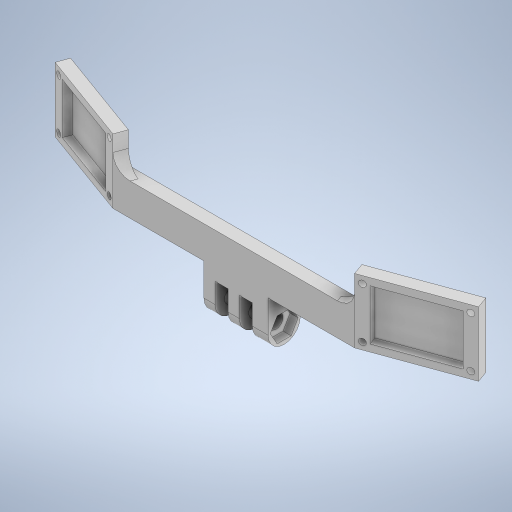
# Autodesk Inventor part: Camera dual mount
Saved by Autodesk Inventor 2024 (Build 280153000, 153)
## iProperties
Created: 2023-07-02
Part Number: Camera dual mount
Material: Generic
Document SubType Name: Modeling
Designer: TEST BENCH
Density: 1 g/cm^3
Appearance: Default
Author: TEST BENCH
Autodesk Inventor part; units mm, degrees
note: some values were not read from the file. Chosen so that the rebuilt part matches the saved one: edges of "Chamfer1".
ref_plane "YZ Plane" through (0, 0, 0) normal (1, 0, 0) x (0, 1, 0)
ref_plane "XZ Plane" through (0, 0, 0) normal (0, 1, 0) x (-1, 0, 0)
ref_plane "XY Plane" through (0, 0, 0) normal (0, 0, 1) x (1, 0, 0)
sketch "Sketch1" plane through (0, 0, 0) normal (0, 0, 1) x (1, 0, 0)
  line L0 (-32.5, 24) -> (32.5, 24)
  line L1 (32.5, 24) -> (32.5, 0)
  line L2 (32.5, 0) -> (-32.5, 0)
  line L3 (-32.5, 0) -> (-32.5, 24)
  point P0 (0, 0)
  dimension "d0" = 0
  dimension "d2" = 65
  dimension "d3" = 32.5
  dimension "d4" = 24
  constraints: 8 end point, 2 parallel, 1 horizontal, 1 perpendicular
  measures "d0" distance from line of L2 point (0, 0)
  measures "d2" distance between parallel lines of L1 L3
  measures "d3" distance from line of point (0, 0) L3
  measures "d4" distance between parallel lines of L2 L0
sketch "Sketch2" plane through (0, 0, 0) normal (0, 1, 0) x (-1, 0, 0)
  line L0 (28.9739, 0) -> (-28.9739, 0) construction
  line L1 (28.9739, 0) -> (51.5266, -8.2085)
  line L2 (51.5266, -8.2085) -> (52.5526, -5.3894)
  line L3 (52.5526, -5.3894) -> (30, 2.8191)
  line L4 (30, 2.8191) -> (28.9739, 0)
  line L5 (-28.9739, 0) -> (-51.5266, -8.2085)
  line L6 (-51.5266, -8.2085) -> (-52.5526, -5.3894)
  line L7 (-52.5526, -5.3894) -> (-30, 2.8191)
  line L8 (-30, 2.8191) -> (-28.9739, 0)
  line L9 (30, 2.8191) -> (-30, 2.8191)
  line L10 (-30, 2.8191) -> (-30, -0.3735)
  line L11 (-30, -0.3735) -> (30, -0.3735)
  line L12 (30, -0.3735) -> (30, 2.8191)
  point P0 (0, 0)
  point P1 (0, 0)
  point P2 (40.2503, -4.1042)
  point P3 (-30, -0.3735)
  dimension "d11" = 160
  dimension "d12" = 160
  dimension "d13" = 0
  dimension "d14" = 0
  dimension "d15" = 3
  dimension "d16" = 24
  dimension "d17" = 24
  dimension "d18" = 3
  dimension "d19" = 0
  dimension "d20" = 60
  constraints: 26 end point, 6 parallel, 3 perpendicular, 2 midpoint, 1 horizontal
  measures "d11" angle of L0 L1
  measures "d12" angle of L5 L0
  measures "d13" distance of point (0, 0) point (0, 0)
  measures "d14" distance of point (0, 0) point (0, 0)
  measures "d15" distance from line of point (40.25, -4.104) L3
  measures "d16" distance of L2.end L3.end
  measures "d17" distance of L6.end L7.end
  measures "d18" distance of L7.end L0.end
  measures "d19" distance from line of L1 L11.end
  measures "d20" distance of L3.end L7.end
extrude "Extrusion1" add sketch "Sketch2" along normal blind 16 contours L4 L12 L1 | L12 L3 L2 L1 | L10 L8 L5 | L5 L6 L7 L10
extrude "Extrusion2" add sketch "Sketch2" along normal blind 8 contours L1 L11 L5 L8 L9 L4
fillet "Fillet1" radius 4 2 edges at (-29.487, 8, 1.4095) (29.487, 8, 1.4095)
sketch "Sketch3" plane through (0, 0, 0) normal (0, -1, 0) x (1, 0, 0)
  line L0 (-25.7433, 2.8191) -> (25.7433, 2.8191) projected
  line L1 (-1.5, 2.8191) -> (1.5, 2.8191)
  line L2 (1.5, 2.8191) -> (1.5, -5.1809)
  line L3 (1.5, -5.1809) -> (-1.5, -5.1809)
  line L4 (-1.5, -5.1809) -> (-1.5, 2.8191)
  line L5 (-4.5, 2.8191) -> (-7.5, 2.8191)
  line L6 (-7.5, 2.8191) -> (-7.5, -5.1809)
  line L7 (-7.5, -5.1809) -> (-4.5, -5.1809)
  line L8 (-4.5, -5.1809) -> (-4.5, 2.8191)
  line L9 (4.5, 2.8191) -> (8.5, 2.8191)
  line L10 (8.5, 2.8191) -> (8.5, -5.1809)
  line L11 (8.5, -5.1809) -> (4.5, -5.1809)
  line L12 (4.5, -5.1809) -> (4.5, 2.8191)
  line L13 (8.5, -5.1809) -> (-7.5, -5.1809)
  line L14 (-7.5, -5.1809) -> (-7.5, 2.8191)
  line L15 (-7.5, 2.8191) -> (8.5, 2.8191)
  line L16 (8.5, 2.8191) -> (8.5, -5.1809)
  line L17 (-1.4, 2.8191) -> (1.4, 2.8191)
  line L18 (1.4, 2.8191) -> (1.4, -5.1809)
  line L19 (1.4, -5.1809) -> (-1.4, -5.1809)
  line L20 (-1.4, -5.1809) -> (-1.4, 2.8191)
  line L21 (-7.4, 2.8191) -> (-4.6, 2.8191)
  line L22 (-4.6, 2.8191) -> (-4.6, -5.1809)
  line L23 (-4.6, -5.1809) -> (-7.4, -5.1809)
  line L24 (-7.4, -5.1809) -> (-7.4, 2.8191)
  line L25 (4.6, 2.8191) -> (8.5, 2.8191)
  line L26 (8.5, 2.8191) -> (8.5, -5.1809)
  line L27 (8.5, -5.1809) -> (4.6, -5.1809)
  line L28 (4.6, -5.1809) -> (4.6, 2.8191)
  line L29 (-7.4, 2.8191) -> (-7.5, 2.8191)
  line L30 (-7.5, 2.8191) -> (-7.5, -5.1809)
  line L31 (-7.5, -5.1809) -> (-7.4, -5.1809)
  line L32 (-7.4, -5.1809) -> (-7.4, 2.8191)
  line L33 (-4.6, 2.8191) -> (-4.5, 2.8191)
  line L34 (-4.5, 2.8191) -> (-4.5, -5.1809)
  line L35 (-4.5, -5.1809) -> (-4.6, -5.1809)
  line L36 (-4.6, -5.1809) -> (-4.6, 2.8191)
  point P0 (0, 0)
  point P1 (0, -5.1809)
  point P2 (0, 2.8191)
  point P3 (-1.5, -1.1809)
  point P4 (4.5, -1.1809)
  point P5 (1.5, 2.8191)
  point P6 (8.5, 2.8191)
  dimension "d26" = 8
  dimension "d27" = 3
  dimension "d28" = 3
  dimension "d29" = 3
  dimension "d30" = 3
  dimension "d31" = 1.5
  dimension "d32" = 4
  dimension "d68" = 2.8
  dimension "d69" = 2.8
  dimension "d70" = 0.1
  dimension "d71" = 0.1
  dimension "d72" = 0.1
  constraints: 72 end point, 18 parallel, 9 horizontal, 9 perpendicular, 9 point on line, 4 midpoint, 1 collinear
  measures "d26" distance of point (0, -5.181) point (0, 2.819)
  measures "d27" distance from line of point (-1.5, -1.181) L2
  measures "d28" distance between parallel lines of L8 L6
  measures "d29" distance between parallel lines of L4 L8
  measures "d30" distance between parallel lines of L12 L2
  measures "d31" distance from line of point (0, 0) L4
  measures "d32" distance from line of point (4.5, -1.181) L10
  measures "d68" distance between parallel lines of L22 L24
  measures "d69" distance between parallel lines of L18 L20
  measures "d70" distance between parallel lines of L14 L24
  measures "d71" distance between parallel lines of L4 L20
  measures "d72" distance between parallel lines of L12 L28
extrude "Extrusion3" add sketch "Sketch3" along normal blind 3 contours L0 L22 L7 L24 | L0 L8 L7 L22 | L0 L4 L13 L8 | L0 L20 L3 L4 | L0 L18 L3 L20 | L0 L2 L3 L18 | L0 L12 L13 L2 | L0 L28 L11 L12 | L0 L10 L11 L28
extrude "Extrusion4" add sketch "Sketch3" along normal blind 12 contours L0 L22 L7 L24 | L0 L18 L3 L20 | L0 L10 L11 L28
fillet "Fillet2" radius 4 6 edges at (6.55, -12, 2.8191) (0, -12, 2.8191) (-6, -12, 2.8191) (-6, -12, -5.1809) (0, -12, -5.1809) (6.55, -12, -5.1809)
chamfer "Chamfer1" distance 4.8075 angle 45 1 edges at (0.55, 0, -0.3735)
sketch "Sketch4" plane through (8.5, 0, 2.8191) normal (1, 0, 0) x (0, 0, -1)
  arc A0 (0, -8) -> (8, -8) centre (4, -8) ccw construction
  line L0 (8, 0) -> (8, -8) construction
  line L1 (0, 0) -> (3.1925, 0) construction
  line L2 (0, 0) -> (0, -8) construction
  line L3 (5.7321, -5) -> (7.4641, -8)
  line L4 (7.4641, -8) -> (5.7321, -11)
  line L5 (5.7321, -11) -> (2.2679, -11)
  line L6 (2.2679, -11) -> (0.5359, -8)
  line L7 (0.5359, -8) -> (2.2679, -5)
  line L8 (2.2679, -5) -> (5.7321, -5)
  line L9 (0, 0) -> (8.2085, 0) construction
  line L10 (3.1925, 4.8075) -> (8, 0) projected
  line L11 (3.1925, 0) -> (3.1925, 4.8075) projected
  point P0 (2.8191, 0)
  point P1 (4, -8)
  point P2 (4, -11)
  point P3 (4, -5)
  point P4 (4, -8)
  dimension "d41" = 6
  constraints: 12 end point, 2 coincident, 2 midpoint, 1 parallel, 13 other
  measures "d41" distance of point (4, -11) point (4, -5)
hole "Hole1" at (8.5, -8, -1.1809) direction (-1, 0, 0) diameter 3.5 end through all
extrude "Extrusion5" cut sketch "Sketch4" against normal blind 2
sketch "Sketch5" plane through (-52.5526, 0, -5.3894) normal (-0.3420201, 0, 0.9396926) x (0.9396926, 0, 0.3420201)
  line L0 (1.5, 14.25) -> (22.5, 14.25) construction
  line L1 (22.5, 14.25) -> (22.5, 1.75) construction
  line L2 (22.5, 1.75) -> (1.5, 1.75) construction
  line L3 (1.5, 1.75) -> (1.5, 14.25) construction
  line L4 (0, 0) -> (24, 0) construction
  line L5 (0, 16) -> (24, 16) construction
  line L6 (0, 0) -> (0, 16) construction
  line L7 (24, 12) -> (24, 16) construction
  line L8 (3, 14.25) -> (21, 14.25)
  line L9 (21, 14.25) -> (21, 1.75)
  line L10 (21, 1.75) -> (3, 1.75)
  line L11 (3, 1.75) -> (3, 14.25)
  point P0 (51.2266, 0)
  dimension "d51" = 21
  dimension "d52" = 12.5
  dimension "d53" = 16
  dimension "d54" = 1.75
  dimension "d55" = 1.5
  dimension "d56" = 24
  dimension "d64" = 18
  dimension "d65" = 3
  constraints: 16 end point, 4 coincident, 4 parallel, 2 horizontal, 2 perpendicular, 2 point on line
  measures "d51" distance of L0.start L0.end
  measures "d52" distance between parallel lines of L2 L0
  measures "d53" distance between parallel lines of L4 L5
  measures "d54" distance between parallel lines of L0 L5
  measures "d55" distance between parallel lines of L6 L3
  measures "d56" distance between parallel lines of L6 L7
  measures "d64" distance between parallel lines of L9 L11
  measures "d65" distance between parallel lines of L6 L11
hole "Hole2" at (-51.1431, 14.25, -4.8764) at (-51.1431, 1.75, -4.8764) at (-31.4095, 1.75, 2.306) at (-31.4095, 14.25, 2.306) direction (0.3420201, 0, -0.9396926) diameter 1.6 end through all
extrude "Extrusion6" cut sketch "Sketch5" against normal blind 2
mirror "Mirror1" about plane through (0, 0, 0) normal (1, 0, 0) of "Hole2", "Extrusion6"
equation "\"d3\" = 0.5 * d2"
equation "\"d12\" = d11"
equation "\"d17\" = d16"
equation "\"d18\" = d15"
equation "\"d28\" = d27"
equation "\"d30\" = d29"
equation "\"d31\" = 0.5 * d27"
equation "\"d69\" = d68"
equation "\"d70\" = -0.5 * d68 + 0.5 * d28"
equation "\"d71\" = d70"
equation "\"d72\" = d70"
equation "\"d54\" = -0.5 * d52 + 0.5 * d53"
equation "\"d55\" = -0.5 * d51 + 0.5 * d56"
equation "\"d65\" = -0.5 * d64 + 0.5 * d56"
body "Solid1"
